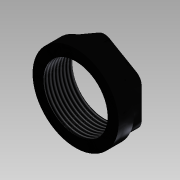
# Autodesk Inventor part: gearProx
Saved by Autodesk Inventor 2015 SP1 (Build 190203100, 203)
## iProperties
Created: 2015-01-28
Part Number: gearProx
Material: Generic
Document SubType Name: Modeling
Designer: Rafi Kurnia Putra
Density: 1 g/cm^3
Appearance: Black
Mass: 1.43462 g
Surface Area: 15.2425 cm^2
Volume: 1.43462 cm^3
Author: Rafi Kurnia Putra
Autodesk Inventor part; units mm, degrees
ref_plane "YZ Plane" through (0, 0, 0) normal (1, 0, 0) x (0, 1, 0)
ref_plane "XZ Plane" through (0, 0, 0) normal (0, 1, 0) x (-1, 0, 0)
ref_plane "XY Plane" through (0, 0, 0) normal (0, 0, 1) x (1, 0, 0)
sketch "Sketch1" plane through (0, 0, 0) normal (0, 1, 0) x (-1, 0, 0)
  circle A0 centre (0, 0) radius 9.2
  circle A1 centre (0, 0) radius 12.35
  dimension "d0" = 18.4
  dimension "d1" = 3.15
  dimension "d9" = 24.7
  constraints: 2 centre point, 1 coincident
  measures "d0" diameter of A0
  measures "d1" radial gap between concentric circles of A0 A1
  measures "d9" diameter of A1
extrude "Extrusion1" add sketch "Sketch1" along normal blind 4.45
thread "Thread1" size "M15x1" class "6H" standard "ANSI Metric M Profile" full length
sketch "Sketch2" plane through (0, 4.45, 0) normal (0, 1, 0) x (1, 0, 0)
  line L0 (-10.6954, 6.175) -> (0, 12.35)
  line L1 (0, 12.35) -> (10.6954, 6.175)
  line L2 (10.6954, 6.175) -> (10.6954, -6.175)
  line L3 (10.6954, -6.175) -> (0, -12.35)
  line L4 (0, -12.35) -> (-10.6954, -6.175)
  line L5 (-10.6954, -6.175) -> (-10.6954, 6.175)
  circle A0 centre (0, 0) radius 9.2
  constraints: 12 end point, 1 centre point, 1 coincident, 1 vertical, 13 other
extrude "Extrusion2" add sketch "Sketch2" along normal blind 3.81
fillet "Fillet1" radius 3 6 edges at (10.6954, 6.355, 6.175) (10.6954, 6.355, -6.175) (0, 6.355, -12.35) (-10.6954, 6.355, -6.175) (-10.6954, 6.355, 6.175) (0, 6.355, 12.35)
body "Solid1"
